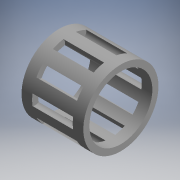
# Autodesk Inventor part: HK0709FMCA
Saved by Autodesk Inventor 2017.3 (Build 213256000, 256)
## iProperties
Part Number: HK0709FMCA
Material: Generic
Catalog Web Link: www.cadenas.de
Description: Needle Roller Shell Bearings open-ended CA-
Vendor: NTN
Document SubType Name: Modeling
Designer: partserver
Manufacturer: NTN
Mass: 0.0983531 g
Surface Area: 4.16382 cm^2
Volume: 0.0983531 cm^3
Density: 1 g/cm^3
Appearance: PSOLRGB-192-192-192
Category: PARTsolutions
Company: NTN
Title: HK0709FMCA
Author: Cadenas PARTsolutions
PSOL_IDENT_0: {$CADENAS_DATA\23d-libs\ntn\needle_roler_bearings\needle_roller_shell_bearings_open_ended_ca.prj},19
PSOL_IDENT_1: 6 {VTYP=3D},{NB=HK0709FMCA},{LINA=HK0709FMCA},{NN=Needle Roller Shell Bearings open-ended CA},{DATE=
PSOL_IDENT_2: 26.11.2019 01:59:50},{GEOMDATE=26.11.2019 00:10:00},{VERSION=},{LINEID=50},{WBVAR=},{WBNUMERIC=}  {N
PSOL_IDENT_3: B=HK0709FMCA},{LINA=HK0709FMCA},{KT=DUMMY},{FW=7},{D=11.0},{C=9},{ORDER=HK0709FM},{CR=3150},{COR=293
PSOL_IDENT_4: 0},{CRF=320},{CORF=299},{LSG=23000},{LSO=34000},{MASS=0.0025},{IT=-},{RT=1.6},{VER=1},{T=0.500},{DW=
PSOL_IDENT_5: 1.500},{LW=5.000},{NR=10.000},{CID=7.750},{CD=9.250},{CW=7.600},{SD=7.350}
NB: HK0709FMCA
NN: Needle Roller Shell Bearings open-ended CA
NBSYN: $ORDER.CA
LINA: HK0709FMCA
CATALOG: NTN Corporation
FW: 7
D: 11
C: 9
ORDER: HK0709FM
CR: 3150
COR: 2930
CRF: 320
CORF: 299
LSG: 23000
LSO: 34000
MASS: 0.0025
IT: -
RT: 1.6
VER: 1
SUPPLIER: NTN
ARTICLENO: HK0709FMCA
BOMINFO: HK0709FMCA
CREATOR: CADENAS GmbH
Autodesk Inventor part; units mm, degrees
ref_plane "YZ Plane" through (0, 0, 0) normal (1, 0, 0) x (0, 1, 0)
ref_plane "XZ Plane" through (0, 0, 0) normal (0, 1, 0) x (-1, 0, 0)
ref_plane "XY Plane" through (0, 0, 0) normal (0, 0, 1) x (1, 0, 0)
sketch "Sketch_1" plane through (0, 0, 0) normal (0, 0, 1) x (1, 0, 0)
  line L0 (8.3, 0) -> (0.7, 0)
  line L1 (0.7, 3.875) -> (8.3, 3.875)
  line L2 (8.3, 3.875) -> (8.3, 4.625)
  line L3 (8.3, 4.625) -> (0.7, 4.625)
  line L4 (0.7, 4.625) -> (0.7, 3.875)
  constraints: 10 end point
revolve "Revolution1" add sketch "Sketch_1" angle 360 about axis through (8.3, 0, 0) along (1, 0, 0)
sketch "Sketch_2" plane through (0, 0, 0) normal (0, 0, 1) x (1, 0, 0)
  line L0 (7, 4.25) -> (2, 4.25)
  line L1 (2, 4.25) -> (2, 5)
  line L2 (2, 5) -> (7, 5)
  line L3 (7, 5) -> (7, 4.25)
  line L4 (7, 4.25) -> (2, 4.25)
  constraints: 10 end point
revolve "Revolution2" cut sketch "Sketch_2" angle 360 about axis through (7, 4.25, 0) along (1, 0, 0)
pattern_circular "Circular Pattern1" count 10 over 360 about axis through (4.5, 0, 0) along (1, 0, 0) of "Revolution2"
ref_plane "IP_1_XY" through (4.5, 0, 0) normal (1, 0, 0) x (0, 0, -1)
ref_plane "IP_1_YZ" through (4.5, 0, 0) normal (0, 0, -1) x (0, 1, 0)
ref_plane "IP_1_ZX" through (4.5, 0, 0) normal (0, 1, 0) x (1, 0, 0)
ref_plane "IP_3_1_XY" through (4.5, 4.25, 0) normal (1, 0, 0) x (0, 0, -1)
ref_plane "IP_3_1_YZ" through (4.5, 4.25, 0) normal (0, 0, -1) x (0, 1, 0)
ref_plane "IP_3_1_ZX" through (4.5, 4.25, 0) normal (0, 1, 0) x (1, 0, 0)
ref_plane "IP_3_10_XY" through (4.5, 3.4383, -2.4981) normal (1, 0, 0) x (0, 0, -1)
ref_plane "IP_3_10_YZ" through (4.5, 3.4383, -2.4981) normal (0, 0, -1) x (0, 1, 0)
ref_plane "IP_3_10_ZX" through (4.5, 3.4383, -2.4981) normal (0, 1, 0) x (1, 0, 0)
ref_plane "IP_3_2_XY" through (4.5, 3.4383, 2.4981) normal (1, 0, 0) x (0, 0, -1)
ref_plane "IP_3_2_YZ" through (4.5, 3.4383, 2.4981) normal (0, 0, -1) x (0, 1, 0)
ref_plane "IP_3_2_ZX" through (4.5, 3.4383, 2.4981) normal (0, 1, 0) x (1, 0, 0)
ref_plane "IP_3_3_XY" through (4.5, 1.3133, 4.042) normal (1, 0, 0) x (0, 0, -1)
ref_plane "IP_3_3_YZ" through (4.5, 1.3133, 4.042) normal (0, 0, -1) x (0, 1, 0)
ref_plane "IP_3_3_ZX" through (4.5, 1.3133, 4.042) normal (0, 1, 0) x (1, 0, 0)
ref_plane "IP_3_4_XY" through (4.5, -1.3133, 4.042) normal (1, 0, 0) x (0, 0, -1)
ref_plane "IP_3_4_YZ" through (4.5, -1.3133, 4.042) normal (0, 0, -1) x (0, 1, 0)
ref_plane "IP_3_4_ZX" through (4.5, -1.3133, 4.042) normal (0, 1, 0) x (1, 0, 0)
ref_plane "IP_3_5_XY" through (4.5, -3.4383, 2.4981) normal (1, 0, 0) x (0, 0, -1)
ref_plane "IP_3_5_YZ" through (4.5, -3.4383, 2.4981) normal (0, 0, -1) x (0, 1, 0)
ref_plane "IP_3_5_ZX" through (4.5, -3.4383, 2.4981) normal (0, 1, 0) x (1, 0, 0)
ref_plane "IP_3_6_XY" through (4.5, -4.25, 0) normal (1, 0, 0) x (0, 0, -1)
ref_plane "IP_3_6_YZ" through (4.5, -4.25, 0) normal (0, 0, -1) x (0, 1, 0)
ref_plane "IP_3_6_ZX" through (4.5, -4.25, 0) normal (0, 1, 0) x (1, 0, 0)
ref_plane "IP_3_7_XY" through (4.5, -3.4383, -2.4981) normal (1, 0, 0) x (0, 0, -1)
ref_plane "IP_3_7_YZ" through (4.5, -3.4383, -2.4981) normal (0, 0, -1) x (0, 1, 0)
ref_plane "IP_3_7_ZX" through (4.5, -3.4383, -2.4981) normal (0, 1, 0) x (1, 0, 0)
ref_plane "IP_3_8_XY" through (4.5, -1.3133, -4.042) normal (1, 0, 0) x (0, 0, -1)
ref_plane "IP_3_8_YZ" through (4.5, -1.3133, -4.042) normal (0, 0, -1) x (0, 1, 0)
ref_plane "IP_3_8_ZX" through (4.5, -1.3133, -4.042) normal (0, 1, 0) x (1, 0, 0)
ref_plane "IP_3_9_XY" through (4.5, 1.3133, -4.042) normal (1, 0, 0) x (0, 0, -1)
ref_plane "IP_3_9_YZ" through (4.5, 1.3133, -4.042) normal (0, 0, -1) x (0, 1, 0)
ref_plane "IP_3_9_ZX" through (4.5, 1.3133, -4.042) normal (0, 1, 0) x (1, 0, 0)
body "Solid1"
